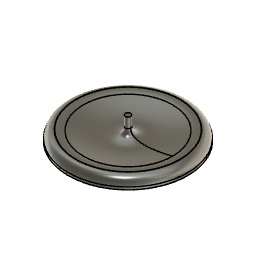
New Base (Autodesk Fusion 360 design; units mm, degrees)
Autodesk Fusion 360 part; units mm, degrees
sketch "Sketch1" plane through (0, 0, 0) normal (0, 1, 0) x (1, 0, 0)
  line L0 (0, 0) -> (30, 0)
  line L1 (30, 0) -> (30, -1.27)
  line L2 (0, 0) -> (0, -11.43)
  line L3 (0, -11.43) -> (1.35, -11.43)
  line L4 (1.35, -11.43) -> (1.35, -6.35)
  spline S0 degree 5 poles (1.35, -6.35) (1.35, -5.9694) (1.4278, -5.2602) (1.778, -4.3531) (2.6877, -3.4451) (4.4374, -2.753) (6.6502, -2.4321) (9.1882, -2.411) (11.9484, -2.6271) (14.8581, -3.0298) (17.5367, -3.5208) (19.6582, -3.9761) (21.1842, -4.334) (22.0932, -4.5575) (22.3741, -4.6275) knots 0 0 0 0 0 0 0.1 0.2 0.3 0.4 0.5 0.6 0.7 0.8 0.9 0.944585 0.944585 0.944585 0.944585 0.944585 0.944585
  line L5 (26.19, -5.08) -> (26.0602, -5.08)
  arc A0 (26.19, -5.08) -> (30, -1.27) centre (26.19, -1.27) ccw
  arc A1 (22.3741, -4.6275) -> (26.0602, -5.08) centre (26.0602, 10.16) ccw
  point P0 (30, -5.08)
  point P1 (6.35, -2.54)
  dimension "d1" = 30
  dimension "d2" = 5.08
  dimension "d3" = 11.43
  dimension "d4" = 1.35
  dimension "d5" = 5.08
  dimension "d6" = 3.81
  dimension "d7" = 15.24
  constraint coincident L0.start L2.start
  constraint horizontal L0
  constraint perpendicular L0 L1
  constraint perpendicular L0 L2
  constraint perpendicular L2 L3
  constraint perpendicular L3 L4
  constraint coincident P0 L5
  constraint coincident P0 L1
  constraint tangent L5 A0
  constraint tangent L1 A0
  constraint tangent S0 A1
  constraint tangent L5 A1
  measures "d1" distance of L0.start L0.end
  measures "d2" distance of L0.end P0
  measures "d3" distance of L0.start L2.end
  measures "d4" distance of L2.end L3.end
  measures "d5" distance of L3.end L4.end
  measures "d6" radius of A0
  measures "d7" radius of A1
revolve "Revolve1" add sketch "Sketch1" angle 360 about axis through (0, 0, 0) along (0, 0, 1)
equation "d4 = 2.7 mm / 2"
